Autodesk Inventor part; units mm, degrees
(part 2 of 2)
sketch "Sketch15" plane through (0, 18, 0) normal (0, 1, 0) x (1, 0, 0)
  arc A0 (330.4278, 208.3333) -> (336.7778, 208.3333) centre (333.6028, 208.3333) ccw projected
  line L0 (330.4278, 208.3333) -> (325.1278, 208.3333) projected
  arc A1 (318.7778, 208.3333) -> (325.1278, 208.3333) centre (321.9528, 208.3333) ccw projected
  line L1 (318.7778, 208.3333) -> (318.7778, 291.6667) projected
  arc A2 (325.1278, 291.6667) -> (318.7778, 291.6667) centre (321.9528, 291.6667) ccw projected
  line L2 (325.1278, 291.6667) -> (330.4278, 291.6667) projected
  arc A3 (336.7778, 291.6667) -> (330.4278, 291.6667) centre (333.6028, 291.6667) ccw projected
  line L3 (336.7778, 291.6667) -> (336.7778, 208.3333) projected
  arc A4 (-336.7778, 208.3333) -> (-330.4278, 208.3333) centre (-333.6028, 208.3333) ccw projected
  line L4 (-336.7778, 208.3333) -> (-336.7778, 291.6667) projected
  arc A5 (-330.4278, 291.6667) -> (-336.7778, 291.6667) centre (-333.6028, 291.6667) ccw projected
  line L5 (-330.4278, 291.6667) -> (-325.1278, 291.6667) projected
  arc A6 (-318.7778, 291.6667) -> (-325.1278, 291.6667) centre (-321.9528, 291.6667) ccw projected
  line L6 (-318.7778, 291.6667) -> (-318.7778, 208.3333) projected
  arc A7 (-325.1278, 208.3333) -> (-318.7778, 208.3333) centre (-321.9528, 208.3333) ccw projected
  line L7 (-325.1278, 208.3333) -> (-330.4278, 208.3333) projected
  line L8 (-205.6667, 75) -> (-205.6667, 116) projected
  line L9 (-205.6667, 116) -> (-246.6667, 116) projected
  line L10 (-246.6667, 116) -> (-246.6667, 134) projected
  line L11 (-246.6667, 134) -> (-205.6667, 134) projected
  line L12 (-205.6667, 134) -> (-205.6667, 175) projected
  line L13 (-205.6667, 175) -> (-187.6667, 175) projected
  line L14 (-187.6667, 175) -> (-187.6667, 134) projected
  line L15 (-187.6667, 134) -> (-146.6667, 134) projected
  line L16 (-146.6667, 134) -> (-146.6667, 116) projected
  line L17 (-146.6667, 116) -> (-187.6667, 116) projected
  line L18 (-187.6667, 116) -> (-187.6667, 75) projected
  line L19 (-187.6667, 75) -> (-205.6667, 75) projected
  line L20 (246.6667, 134) -> (246.6667, 116) projected
  line L21 (246.6667, 116) -> (205.6667, 116) projected
  line L22 (205.6667, 116) -> (205.6667, 75) projected
  line L23 (205.6667, 75) -> (187.6667, 75) projected
  line L24 (187.6667, 75) -> (187.6667, 116) projected
  line L25 (187.6667, 116) -> (146.6667, 116) projected
  line L26 (146.6667, 116) -> (146.6667, 134) projected
  line L27 (146.6667, 134) -> (187.6667, 134) projected
  line L28 (187.6667, 134) -> (187.6667, 175) projected
  line L29 (187.6667, 175) -> (205.6667, 175) projected
  line L30 (205.6667, 175) -> (205.6667, 134) projected
  line L31 (205.6667, 134) -> (246.6667, 134) projected
  line L32 (-246.6667, -134) -> (-246.6667, -116) projected
  line L33 (-246.6667, -116) -> (-205.6667, -116) projected
  line L34 (-205.6667, -116) -> (-205.6667, -75) projected
  line L35 (-205.6667, -75) -> (-187.6667, -75) projected
  line L36 (-187.6667, -75) -> (-187.6667, -116) projected
  line L37 (-187.6667, -116) -> (-146.6667, -116) projected
  line L38 (-146.6667, -116) -> (-146.6667, -134) projected
  line L39 (-146.6667, -134) -> (-187.6667, -134) projected
  line L40 (-187.6667, -134) -> (-187.6667, -175) projected
  line L41 (-187.6667, -175) -> (-205.6667, -175) projected
  line L42 (-205.6667, -175) -> (-205.6667, -134) projected
  line L43 (-205.6667, -134) -> (-246.6667, -134) projected
  line L44 (246.6667, -116) -> (246.6667, -134) projected
  line L45 (246.6667, -134) -> (205.6667, -134) projected
  line L46 (205.6667, -134) -> (205.6667, -175) projected
  line L47 (205.6667, -175) -> (187.6667, -175) projected
  line L48 (187.6667, -175) -> (187.6667, -134) projected
  line L49 (187.6667, -134) -> (146.6667, -134) projected
  line L50 (146.6667, -134) -> (146.6667, -116) projected
  line L51 (146.6667, -116) -> (187.6667, -116) projected
  line L52 (187.6667, -116) -> (187.6667, -75) projected
  line L53 (187.6667, -75) -> (205.6667, -75) projected
  line L54 (205.6667, -75) -> (205.6667, -116) projected
  line L55 (205.6667, -116) -> (246.6667, -116) projected
  arc A8 (572, 214.6833) -> (572, 208.3333) centre (572, 211.5083) ccw projected
  line L56 (572, 214.6833) -> (572, 285.3167) projected
  arc A9 (572, 291.6667) -> (572, 285.3167) centre (572, 288.4917) ccw projected
  line L57 (572, 291.6667) -> (590, 291.6667) projected
  line L58 (590, 291.6667) -> (590, 375) projected
  line L59 (590, 375) -> (246.6667, 375) projected
  line L60 (246.6667, 375) -> (246.6667, 357) projected
  arc A10 (240.3167, 357) -> (246.6667, 357) centre (243.4917, 357) ccw projected
  line L61 (240.3167, 357) -> (205.6667, 357) projected
  line L62 (205.6667, 357) -> (205.6667, 322.35) projected
  arc A11 (205.6667, 316) -> (205.6667, 322.35) centre (205.6667, 319.175) ccw projected
  line L63 (205.6667, 316) -> (187.6667, 316) projected
  arc A12 (187.6667, 322.35) -> (187.6667, 316) centre (187.6667, 319.175) ccw projected
  line L64 (187.6667, 322.35) -> (187.6667, 357) projected
  line L65 (187.6667, 357) -> (153.0167, 357) projected
  arc A13 (146.6667, 357) -> (153.0167, 357) centre (149.8417, 357) ccw projected
  line L66 (146.6667, 357) -> (146.6667, 375) projected
  line L67 (146.6667, 375) -> (-146.6667, 375) projected
  line L68 (-146.6667, 375) -> (-146.6667, 357) projected
  arc A14 (-153.0167, 357) -> (-146.6667, 357) centre (-149.8417, 357) ccw projected
  line L69 (-153.0167, 357) -> (-187.6667, 357) projected
  line L70 (-187.6667, 357) -> (-187.6667, 322.35) projected
  arc A15 (-187.6667, 316) -> (-187.6667, 322.35) centre (-187.6667, 319.175) ccw projected
  line L71 (-187.6667, 316) -> (-205.6667, 316) projected
  arc A16 (-205.6667, 322.35) -> (-205.6667, 316) centre (-205.6667, 319.175) ccw projected
  line L72 (-205.6667, 322.35) -> (-205.6667, 357) projected
  line L73 (-205.6667, 357) -> (-240.3167, 357) projected
  arc A17 (-246.6667, 357) -> (-240.3167, 357) centre (-243.4917, 357) ccw projected
  line L74 (-246.6667, 357) -> (-246.6667, 375) projected
  line L75 (-246.6667, 375) -> (-590, 375) projected
  line L76 (-590, 375) -> (-590, 291.6667) projected
  line L77 (-590, 291.6667) -> (-572, 291.6667) projected
  arc A18 (-572, 285.3167) -> (-572, 291.6667) centre (-572, 288.4917) ccw projected
  line L78 (-572, 285.3167) -> (-572, 214.6833) projected
  arc A19 (-572, 208.3333) -> (-572, 214.6833) centre (-572, 211.5083) ccw projected
  line L79 (-572, 208.3333) -> (-590, 208.3333) projected
  line L80 (-590, 208.3333) -> (-590, 175) projected
  line L81 (-590, 175) -> (-572, 175) projected
  arc A20 (-572, 168.65) -> (-572, 175) centre (-572, 171.825) ccw projected
  line L82 (-572, 168.65) -> (-572, 134) projected
  line L83 (-572, 134) -> (-537.35, 134) projected
  arc A21 (-531, 134) -> (-537.35, 134) centre (-534.175, 134) ccw projected
  line L84 (-531, 134) -> (-531, 116) projected
  arc A22 (-537.35, 116) -> (-531, 116) centre (-534.175, 116) ccw projected
  line L85 (-537.35, 116) -> (-572, 116) projected
  line L86 (-572, 116) -> (-572, 81.35) projected
  arc A23 (-572, 75) -> (-572, 81.35) centre (-572, 78.175) ccw projected
  line L87 (-572, 75) -> (-590, 75) projected
  line L88 (-590, 75) -> (-590, -75) projected
  line L89 (-590, -75) -> (-572, -75) projected
  arc A24 (-572, -81.35) -> (-572, -75) centre (-572, -78.175) ccw projected
  line L90 (-572, -81.35) -> (-572, -116) projected
  line L91 (-572, -116) -> (-537.35, -116) projected
  arc A25 (-531, -116) -> (-537.35, -116) centre (-534.175, -116) ccw projected
  line L92 (-531, -116) -> (-531, -134) projected
  arc A26 (-537.35, -134) -> (-531, -134) centre (-534.175, -134) ccw projected
  line L93 (-537.35, -134) -> (-572, -134) projected
  line L94 (-572, -134) -> (-572, -168.65) projected
  arc A27 (-572, -175) -> (-572, -168.65) centre (-572, -171.825) ccw projected
  line L95 (-572, -175) -> (-590, -175) projected
  line L96 (-590, -175) -> (-590, -375) projected
  line L97 (-590, -375) -> (-246.6667, -375) projected
  line L98 (-246.6667, -375) -> (-246.6667, -357) projected
  arc A28 (-240.3167, -357) -> (-246.6667, -357) centre (-243.4917, -357) ccw projected
  line L99 (-240.3167, -357) -> (-205.6667, -357) projected
  line L100 (-205.6667, -357) -> (-205.6667, -322.35) projected
  arc A29 (-205.6667, -316) -> (-205.6667, -322.35) centre (-205.6667, -319.175) ccw projected
  line L101 (-205.6667, -316) -> (-187.6667, -316) projected
  arc A30 (-187.6667, -322.35) -> (-187.6667, -316) centre (-187.6667, -319.175) ccw projected
  line L102 (-187.6667, -322.35) -> (-187.6667, -357) projected
  line L103 (-187.6667, -357) -> (-153.0167, -357) projected
  arc A31 (-146.6667, -357) -> (-153.0167, -357) centre (-149.8417, -357) ccw projected
  line L104 (-146.6667, -357) -> (-146.6667, -375) projected
  line L105 (-146.6667, -375) -> (146.6667, -375) projected
  line L106 (146.6667, -375) -> (146.6667, -357) projected
  arc A32 (153.0167, -357) -> (146.6667, -357) centre (149.8417, -357) ccw projected
  line L107 (153.0167, -357) -> (187.6667, -357) projected
  line L108 (187.6667, -357) -> (187.6667, -322.35) projected
  arc A33 (187.6667, -316) -> (187.6667, -322.35) centre (187.6667, -319.175) ccw projected
  line L109 (187.6667, -316) -> (205.6667, -316) projected
  arc A34 (205.6667, -322.35) -> (205.6667, -316) centre (205.6667, -319.175) ccw projected
  line L110 (205.6667, -322.35) -> (205.6667, -357) projected
  line L111 (205.6667, -357) -> (240.3167, -357) projected
  arc A35 (246.6667, -357) -> (240.3167, -357) centre (243.4917, -357) ccw projected
  line L112 (246.6667, -357) -> (246.6667, -375) projected
  line L113 (246.6667, -375) -> (590, -375) projected
  line L114 (590, -375) -> (590, -175) projected
  line L115 (590, -175) -> (572, -175) projected
  arc A36 (572, -168.65) -> (572, -175) centre (572, -171.825) ccw projected
  line L116 (572, -168.65) -> (572, -134) projected
  line L117 (572, -134) -> (537.35, -134) projected
  arc A37 (531, -134) -> (537.35, -134) centre (534.175, -134) ccw projected
  line L118 (531, -134) -> (531, -116) projected
  arc A38 (537.35, -116) -> (531, -116) centre (534.175, -116) ccw projected
  line L119 (537.35, -116) -> (572, -116) projected
  line L120 (572, -116) -> (572, -81.35) projected
  arc A39 (572, -75) -> (572, -81.35) centre (572, -78.175) ccw projected
  line L121 (572, -75) -> (590, -75) projected
  line L122 (590, -75) -> (590, 75) projected
  line L123 (590, 75) -> (572, 75) projected
  arc A40 (572, 81.35) -> (572, 75) centre (572, 78.175) ccw projected
  line L124 (572, 81.35) -> (572, 116) projected
  line L125 (572, 116) -> (537.35, 116) projected
  arc A41 (531, 116) -> (537.35, 116) centre (534.175, 116) ccw projected
  line L126 (531, 116) -> (531, 134) projected
  arc A42 (537.35, 134) -> (531, 134) centre (534.175, 134) ccw projected
  line L127 (537.35, 134) -> (572, 134) projected
  line L128 (572, 134) -> (572, 168.65) projected
  arc A43 (572, 175) -> (572, 168.65) centre (572, 171.825) ccw projected
  line L129 (572, 175) -> (590, 175) projected
  line L130 (590, 175) -> (590, 208.3333) projected
  line L131 (590, 208.3333) -> (572, 208.3333) projected
  point P0 (0, 0)
  point P1 (-205.6667, 171.825)
  point P2 (-243.4917, 134)
  dimension "d79" = 3.175
  dimension "d80" = 3.175
  constraints: 1 horizontal alignment, 1 vertical alignment
  measures "d79" distance from line of L10 point (-243.492, 134)
  measures "d80" distance from line of L13 point (-205.667, 171.825)
hole "Hole5" at (-205.6667, 18, -171.825) at (-243.4917, 18, -134) direction (0, -1, 0) diameter 6.35 end through all
mirror "Mirror21" about plane through (-196.6667, 0, -357) normal (1, 0, 0) of "Hole5"
mirror "Mirror22" about plane through (-572, 0, -125) normal (0, 0, 1) of "Hole5", "Mirror21"
mirror "Mirror23" about plane through (-590, 0, 0) normal (0, 0, 1) of "Hole5", "Mirror21", "Mirror22"
mirror "Mirror24" about plane through (0, 0, 375) normal (-1, 0, 0) of "Hole5", "Mirror21", "Mirror22", "Mirror23"
sketch "Sketch16" plane through (0, 18, 0) normal (0, 1, 0) x (1, 0, 0)
  arc A0 (-572, 214.6833) -> (-572, 208.3333) centre (-572, 211.5083) ccw projected
  line L0 (-572, 285.3167) -> (-572, 214.6833) projected
  arc A1 (-572, 291.6667) -> (-572, 285.3167) centre (-572, 288.4917) ccw projected
  line L1 (-590, 291.6667) -> (-572, 291.6667) projected
  line L2 (-590, 208.3333) -> (-590, 291.6667) projected
  line L3 (-572, 208.3333) -> (-590, 208.3333) projected
  point P0 (0, 0)
  point P1 (-581, 250)
  point P2 (-590, 250)
  dimension "d89" = 9
  constraints: 1 horizontal alignment, 1 midpoint
  measures "d89" distance of point (-590, 250) point (-581, 250)
hole "Hole6" at (-581, 18, -250) direction (0, -1, 0) diameter 6.35 end through all
mirror "Mirror25" about plane through (0, 0, 375) normal (-1, 0, 0) of "Hole6"
fillet "Fillet1" radius 3.175 16 edges at (-246.6667, 9, 375) (-146.6667, 9, 375) (146.6667, 9, 375) (246.6667, 9, 375) (590, 9, 75) (590, 9, 175) (590, 9, -75) (590, 9, -175) (146.6667, 9, -375) (246.6667, 9, -375) (-246.6667, 9, -375) (-146.6667, 9, -375) (-590, 9, -175) (-590, 9, -75) (-590, 9, 75) (-590, 9, 175)
equation "\"d0\" = tableLength"
equation "\"d1\" = tableWidth"
equation "\"d2\" = plyThickness"
equation "\"d4\" = plyThickness"
equation "\"d5\" = legTabTotalWidth"
equation "\"d6\" = 0.333333 * tableWidth"
equation "\"d7\" = plyThickness"
equation "\"d22\" = plyThickness"
equation "\"d23\" = 0.5 * plyThickness + 0.5 * legTabTotalWidth"
equation "\"d24\" = plyThickness"
equation "\"d9\" = plyThickness"
equation "\"d10\" = legTabTotalWidth"
equation "\"d11\" = 0.333333 * tableLength"
equation "\"d12\" = plyThickness"
equation "\"d26\" = plyThickness"
equation "\"d27\" = 0.5 * plyThickness + 0.5 * legTabTotalWidth"
equation "\"d28\" = plyThickness"
equation "\"d14\" = plyThickness"
equation "\"d15\" = legTabTotalWidth"
equation "\"d16\" = plyThickness"
equation "\"d18\" = plyThickness"
equation "\"d19\" = legTabTotalWidth"
equation "\"d20\" = plyThickness"
equation "\"d30\" = shelfWidth"
equation "\"d31\" = shelfLength"
equation "\"d32\" = plyThickness"
equation "\"d33\" = 0.333333 * shelfWidth"
equation "\"d36\" = 0.333333 * shelfWidth"
equation "\"d37\" = plyThickness"
equation "\"d38\" = 0.5 * plyThickness"
equation "\"d39\" = 0.222222 * shelfLength"
equation "\"d40\" = 0.5 * plyThickness"
equation "\"d42\" = 0.5 * plyThickness"
equation "\"d44\" = 0.5 * millDiameter"
equation "\"d45\" = 0.5 * millDiameter"
equation "\"d46\" = millDiameter"
equation "\"d53\" = 0.5 * millDiameter"
equation "\"d54\" = 0.5 * millDiameter"
equation "\"d55\" = millDiameter"
equation "\"d62\" = 0.5 * millDiameter"
equation "\"d63\" = millDiameter"
equation "\"d68\" = 0.5 * plyThickness"
equation "\"d70\" = 0.5 * millDiameter"
equation "\"d71\" = 0.5 * millDiameter"
equation "\"d72\" = millDiameter"
equation "\"d77\" = 0.5 * plyThickness"
equation "\"d79\" = 0.5 * millDiameter"
equation "\"d80\" = 0.5 * millDiameter"
equation "\"d81\" = millDiameter"
equation "\"d86\" = 0.5 * plyThickness"
equation "\"d89\" = 0.5 * plyThickness"
equation "\"d90\" = millDiameter"
equation "\"d95\" = 0.5 * plyThickness"
equation "\"plyThickness\" = 18"
equation "\"legHeight\" = 702"
equation "\"tableLength\" = 1180"
equation "\"tableWidth\" = 750"
equation "\"millDiameter\" = 6.35"
equation "\"legTopTabHeight\" = 18"
equation "\"legTabTotalWidth\" = 100"
equation "\"legTopSlotDepth\" = 49"
equation "\"shelfWidth\" = 250"
equation "\"shelfLength\" = 1180"
body "Solid1"
